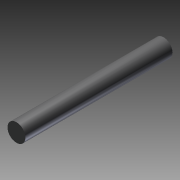
# Autodesk Inventor part: SHHPS5-2-r
Saved by Autodesk Inventor 2015 SP1 (Build 190203100, 203)
## iProperties
Category: PARTsolutions
Company: MISUMI
Created: 2015-01-26
Part Number: SHHPS5-2-r
Catalog Web Link: www.cadenas.de
Description: SHHPS,SHHPSD, SHHPT-r-Stainless Steel Hinges, Steel Hinges
Vendor: MISUMI
Document SubType Name: Modeling
Designer: PARTuser1
Manufacturer: MISUMI
Mass: 0.805033 g
Surface Area: 6.83296 cm^2
Volume: 0.805033 cm^3
Density: 1 g/cm^3
Material: Generic
Appearance: PSOLRGB-192-192-192
PSOL_IDENT_0: {\\10.0.0.236\data_v8\23d-libs\misumi\metric\39_accessories_for_al_extrusions\shhps_pin.prj},188 {VT
PSOL_IDENT_1: YP=3D},{NB=SHHPS5-2-r},{LINA=SHHPS5-2-r},{NN=SHHPS,SHHPSD, SHHPT-r},{DATE=17.11.2014 05:31:34},{GEOM
PSOL_IDENT_2: DATE=13.05.2009 09:09:00},{VERSION=},{LINEID=10},{LINESUBID=-1},{WBVAR=TS,NOH,ALT1}  {NB=SHHPS5-2-r}
PSOL_IDENT_3: ,{LINA=SHHPS5-2-r},{KT=DUMMY},{PN=SHHPS5-2},{TYPE=SHHPS},{TS=1},{MAT=316 Stainless Steel},{ST=-},{NO=
PSOL_IDENT_4: 5},{NOH=2},{ALKG=9},{ALN=88},{MASS=43},{L=41},{W=36},{K=8.0},{P=25},{J=7.5},{S=21},{ND=5.5},{NC=0.0}
PSOL_IDENT_5: ,{T=2.0},{E=4.6},{R=4.6},{CR=7.5},{D=5},{AB=CBSST5-8},{QB=4},{ALT1=},{TIF=1},{M=5},{L1=8},{MAT1=SUSX
PSOL_IDENT_6: M7(30430 Stainless Steel)},{NO1=5},{MAT2=316 Stainless Steel (or Equivalent)},{M1=4},{L2=8},{MAT3=SU
PSOL_IDENT_7: S304(304 Stainless Steel)(1.4301_X5CrNi18-10)}
SUPPLIER: MISUMI
ARTICLENO: SHHPS5-2-r
BOMINFO: SHHPS5-2-r
CREATOR: CADENAS GmbH
Title: Hinge Pin
Author: Misumi
Comments: Stainless Steel Hinges, Steel Hinges
Autodesk Inventor part; units mm, degrees
sketch "Sketch_1" plane through (0, 0, 0) normal (0, 0, 1) x (1, 0, 0)
  line L0 (0, -20.5) -> (0, 20.5)
  line L1 (0, 20.5) -> (2.5, 20.5)
  line L2 (2.5, 20.5) -> (2.5, -20.5)
  line L3 (2.5, -20.5) -> (0, -20.5)
  line L4 (0, -20.5) -> (0, 20.5)
  constraints: 10 end point
revolve "Revolution1" add sketch "Sketch_1" angle 360 about axis through (0, -20.5, 0) along (0, -1, 0)
ref_plane "pin_XY" through (0, 0, 0) normal (0, 1, 0) x (1, 0, 0)
ref_plane "pin_YZ" through (0, 0, 0) normal (1, 0, 0) x (0, 0, -1)
ref_plane "pin_ZX" through (0, 0, 0) normal (0, 0, -1) x (0, 1, 0)
body "Solid1"
